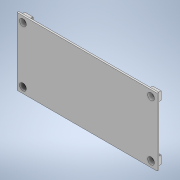
# Autodesk Inventor part: TimDeckel
Saved by Autodesk Inventor 2022 (Build 260153000, 153)
## iProperties
Created: 2023-01-01
Part Number: TimDeckel
Material: Generisch
Document SubType Name: Modeling
Designer: Joshua
Density: 1 g/cm^3
Appearance: Vorgabe
Author: Joshua
Autodesk Inventor part; units mm, degrees
ref_plane "YZ Plane" through (0, 0, 0) normal (1, 0, 0) x (0, 1, 0)
ref_plane "XZ Plane" through (0, 0, 0) normal (0, 1, 0) x (-1, 0, 0)
ref_plane "XY Plane" through (0, 0, 0) normal (0, 0, 1) x (1, 0, 0)
sketch "Skizze1" plane through (0, 0, 0) normal (0, 0, 1) x (1, 0, 0)
  line L0 (0, 0) -> (166, 0)
  line L1 (166, 0) -> (166, 80)
  line L2 (166, 80) -> (0, 80)
  line L3 (0, 80) -> (0, 0)
  dimension "d0" = 80
  dimension "d1" = 166
  constraints: 8 end point, 2 parallel, 1 horizontal, 1 perpendicular
  measures "d0" distance of L2.end L0.start
  measures "d1" distance of L1.end L2.end
extrude "Extrusion1" add sketch "Skizze1" along normal blind 2
sketch "Skizze2" plane through (0, 0, 0) normal (0, 0, -1) x (-1, 0, 0)
  line L0 (-2.2, 77.8) -> (-12, 77.8)
  line L1 (-12, 77.8) -> (-12, 68)
  line L2 (-12, 68) -> (-2.2, 68)
  line L3 (-2.2, 68) -> (-2.2, 77.8)
  line L4 (0, 80) -> (0, 0) projected
  line L5 (-166, 80) -> (0, 80) projected
  line L6 (0, 80) -> (0, 0) projected
  line L7 (0, 40) -> (18.01, 40)
  line L8 (-166, 80) -> (0, 80) projected
  line L9 (-83, 80) -> (-83, 127.491)
  line L10 (-2.2, 2.2) -> (-12, 2.2)
  line L11 (-12, 2.2) -> (-12, 12)
  line L12 (-12, 12) -> (-2.2, 12)
  line L13 (-2.2, 12) -> (-2.2, 2.2)
  line L14 (-163.8, 77.8) -> (-154, 77.8)
  line L15 (-154, 77.8) -> (-154, 68)
  line L16 (-154, 68) -> (-163.8, 68)
  line L17 (-163.8, 68) -> (-163.8, 77.8)
  line L18 (-166, 80) -> (-166, 0)
  line L19 (-166, 80) -> (-166, 0)
  line L20 (-163.8, 2.2) -> (-154, 2.2)
  line L21 (-154, 2.2) -> (-154, 12)
  line L22 (-154, 12) -> (-163.8, 12)
  line L23 (-163.8, 12) -> (-163.8, 2.2)
  point P0 (-166, 40)
  dimension "d4" = 2.2
  dimension "d5" = 2.2
  dimension "d6" = 9.8
  dimension "d7" = 9.8
  dimension "d8" = 40
  constraints: 40 end point, 14 symmetric about line, 3 midpoint, 2 horizontal, 2 parallel, 1 perpendicular, 1 vertical
  measures "d4" distance between parallel lines of L3 L4
  measures "d5" distance between parallel lines of L5 L0
  measures "d6" distance of L2.end L0.start
  measures "d7" distance of L1.end L2.end
  measures "d8" distance between parallel lines of L5 L7
extrude "Extrusion2" add sketch "Skizze2" along normal blind 5
sketch "Skizze3" plane through (0, 0, 2) normal (0, 0, 1) x (1, 0, 0)
  line L0 (0, 80) -> (0, 0) projected
  line L1 (0, 0) -> (166, 0) projected
  line L2 (0, 80) -> (0, 0) projected
  line L3 (0, 40) -> (-51.158, 40)
  line L4 (0, 0) -> (166, 0) projected
  line L5 (83, 0) -> (83, -45.9243)
  line L6 (166, 80) -> (166, 0)
  line L7 (166, 0) -> (0, 0)
  line L8 (166, 80) -> (166, 0)
  line L9 (166, 40) -> (217.158, 40)
  line L10 (166, 0) -> (0, 0)
  point P0 (7, 7)
  point P1 (7, 73)
  point P2 (159, 7)
  point P3 (159, 73)
  dimension "d11" = 7
  dimension "d12" = 7
  constraints: 14 end point, 8 symmetric about line, 2 midpoint, 1 horizontal, 1 vertical
  measures "d11" distance from line of L0 point (7, 7)
  measures "d12" distance from line of L1 point (7, 7)
hole "Bohrung1" at (7, 7, 2) at (7, 73, 2) at (159, 73, 2) at (159, 7, 2) direction (0, 0, -1) diameter 3.5 depth 8 tip angle 118
sketch "Skizze4" plane through (0, 0, 2) normal (0, 0, 1) x (1, 0, 0)
  circle A0 centre (7, 7) radius 1.75 projected
  circle A1 centre (7, 73) radius 1.75 projected
  circle A2 centre (159, 7) radius 1.75 projected
  circle A3 centre (159, 73) radius 1.75 projected
  point P0 (0, 0)
  constraints: 4 coincident
hole "Bohrung2" at (7, 7, 2) at (7, 73, 2) at (159, 7, 2) at (159, 73, 2) direction (0, 0, -1) diameter 8 depth 5 tip angle 118
